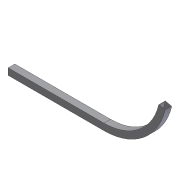
# Autodesk Inventor part: Frame_RearBallGuide
Saved by Autodesk Inventor 2012 (Build 160160000, 160)
## iProperties
Created: 2012-01-11
Part Number: Frame_RearBallGuide
Material: Default
Document SubType Name: Modeling
Designer: JesseK
Density: 1 g/cm^3
Author: JesseK
Autodesk Inventor part; units mm, degrees
ref_plane "YZ Plane" through (0, 0, 0) normal (1, 0, 0) x (0, 1, 0)
ref_plane "XZ Plane" through (0, 0, 0) normal (0, 1, 0) x (-1, 0, 0)
ref_plane "XY Plane" through (0, 0, 0) normal (0, 0, 1) x (1, 0, 0)
sketch "Sketch1" plane through (0, 0, 0) normal (0, 0, 1) x (1, 0, 0)
  arc A0 (368.3, 25.4) -> (578.4957, 191.999) centre (368.3, 241.3) ccw
  arc A1 (368.3, 0) -> (603.2246, 186.1989) centre (368.3, 241.3) ccw
  line L0 (368.3, 25.4) -> (0, 25.4)
  line L1 (0, 25.4) -> (0, 0)
  line L2 (0, 0) -> (368.3, 0)
  line L3 (578.4957, 191.999) -> (603.2246, 186.1989)
  line L4 (368.3, 25.4) -> (368.3, 241.3) construction
  line L5 (368.3, 241.3) -> (578.4957, 191.999) construction
  dimension "d5" = 25.4
  dimension "d6" = 215.9
  dimension "d7" = 368.3
  dimension "d8" = 76.8
  constraints: 12 end point, 4 point on circle, 2 centre point, 2 horizontal, 2 tangent, 2 vertical, 1 coincident, 1 collinear
  measures "d5" distance of L0.end L1.end
  measures "d6" radius of A0
  measures "d7" distance of L0.start L0.end
  measures "d8" angle of L5 L4
extrude "Extrusion1" add sketch "Sketch1" along normal blind 25.4
shell "Shell1" thickness 1.5875 removed faces 2 at (0, 8.4667, 8.4667) at (586.7387, 190.0657, 16.9333)
body "Solid1"
